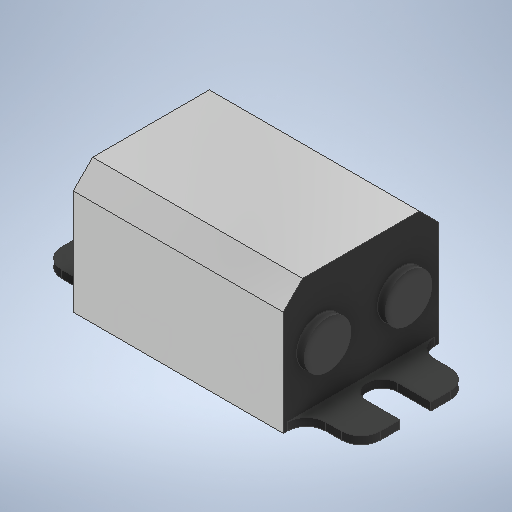
# Autodesk Inventor part: 5vconverter
Saved by Autodesk Inventor 2025 (Build 290162000, 162)
## iProperties
Created: 2025-05-12
Part Number: 5vconverter
Material: Generic
Document SubType Name: Modeling
Designer: ethan
Density: 1 g/cm^3
Appearance: Default
Author: ethan
Autodesk Inventor part; units mm, degrees
ref_plane "YZ Plane" through (0, 0, 0) normal (1, 0, 0) x (0, 1, 0)
ref_plane "XZ Plane" through (0, 0, 0) normal (0, 1, 0) x (-1, 0, 0)
sketch "Sketch1" plane through (0, 0, 0) normal (0, 1, 0) x (-1, 0, 0)
  line L0 (-17.145, 12.7) -> (17.145, 12.7)
  line L1 (17.145, 12.7) -> (17.145, -12.7)
  line L2 (17.145, -12.7) -> (-17.145, -12.7)
  line L3 (-17.145, -12.7) -> (-17.145, 12.7)
  line L4 (-17.145, 12.7) -> (17.145, -12.7) construction
  line L5 (17.145, 12.7) -> (-17.145, -12.7) construction
  point P0 (0, 0)
  dimension "d0" = 34.29
  dimension "d1" = 25.4
  constraints: 12 end point, 2 midpoint, 2 parallel, 1 horizontal, 1 perpendicular
  measures "d0" distance of L1.end L2.end
  measures "d1" distance of L0.end L1.end
extrude "Extrusion1" add sketch "Sketch1" along normal blind 20.32
sketch "Sketch2" plane through (17.145, 0, 12.7) normal (1, 0, 0) x (0, 0, -1)
  line L0 (0, 0) -> (25.4, 0) projected
  line L1 (25.4, 0) -> (25.4, 20.32) projected
  line L2 (0, 20.32) -> (25.4, 20.32) projected
  line L3 (0, 0) -> (0, 20.32) projected
  circle A0 centre (19.2135, 10.16) radius 3.81
  circle A1 centre (5.9899, 10.16) radius 3.81
  point P0 (12.7, 0)
  dimension "d4" = 7.62
  dimension "d5" = 7.62
  constraints: 2 centre point
  measures "d4" diameter of A0
  measures "d5" diameter of A1
ref_plane "Work Plane1" through (0, 0, 12.7) normal (1, 0, 0) x (0, 0, -1)
extrude "Extrusion2" add sketch "Sketch2" along normal blind 1.27 separate body contours A0 | A1
mirror "Mirror1" about plane through (0, 0, 12.7) normal (1, 0, 0) of "Extrusion2" bodies 2
sketch "Sketch3" plane through (0, 0, 0) normal (0, -1, 0) x (1, 0, 0)
  line L0 (17.145, -12.7) -> (-17.145, -12.7) projected
  line L1 (17.145, 12.7) -> (17.145, -12.7) projected
  line L2 (-17.145, 12.7) -> (17.145, 12.7) projected
  line L3 (-17.145, -12.7) -> (-17.145, 12.7) projected
  line L4 (16.1925, 2.54) -> (18.0975, 2.54)
  line L5 (18.0975, 2.54) -> (18.0975, 0)
  line L6 (18.0975, -2.54) -> (16.1925, -2.54)
  line L7 (16.1925, -2.54) -> (16.1925, 2.54)
  line L8 (16.1925, 2.54) -> (18.0975, -2.54) construction
  line L9 (18.0975, 2.54) -> (16.1925, -2.54) construction
  line L10 (20.6375, -2.54) -> (26.035, -2.54)
  line L11 (26.035, -2.54) -> (26.035, -5.715)
  line L12 (22.86, -8.89) -> (20.32, -8.89)
  arc A0 (22.86, -8.89) -> (26.035, -5.715) centre (22.86, -5.715) ccw
  arc A1 (18.0975, 0) -> (20.6375, -2.54) centre (20.6375, 0) ccw
  line L13 (22.86, 0) -> (28.1937, 0)
  line L14 (17.145, 12.7) -> (-17.145, 12.7)
  line L15 (17.145, -12.7) -> (17.145, -12.065)
  line L16 (18.0975, 2.54) -> (16.1925, 2.54)
  line L17 (16.1925, 2.54) -> (16.1925, -2.54)
  line L18 (16.1925, -2.54) -> (18.0975, 2.54) construction
  line L19 (18.0975, -2.54) -> (16.1925, 2.54) construction
  line L20 (20.6375, 2.54) -> (26.035, 2.54)
  line L21 (26.035, 2.54) -> (26.035, 5.715)
  line L22 (22.86, 8.89) -> (20.32, 8.89)
  arc A2 (26.035, 5.715) -> (22.86, 8.89) centre (22.86, 5.715) ccw
  arc A3 (20.6375, 2.54) -> (18.0975, 0) centre (20.6375, 0) ccw
  arc A4 (20.32, -8.89) -> (17.145, -12.065) centre (20.32, -12.065) ccw
  line L23 (17.145, 12.7) -> (17.145, 12.065)
  arc A5 (17.145, 12.065) -> (20.32, 8.89) centre (20.32, 12.065) ccw
  point P0 (0, 0)
  point P1 (17.145, 0)
  point P2 (17.145, -2.54)
  point P3 (26.035, -8.89)
  point P4 (17.145, -8.89)
  point P5 (17.145, 2.54)
  point P6 (26.035, 8.89)
  point P7 (17.145, 8.89)
  dimension "d8" = 1.905
  dimension "d9" = 5.08
  dimension "d10" = 8.89
  dimension "d11" = 6.35
  dimension "d12" = 3.175
  dimension "d13" = 2.54
  dimension "d14" = 3.175
  dimension "d15" = 3.175
  constraints: 40 end point, 15 point on line, 14 symmetric about line, 12 point on circle, 8 tangent, 6 centre point, 4 midpoint, 2 horizontal, 2 parallel, 2 perpendicular, 1 collinear, 1 vertical, 2 other
  measures "d8" distance of L6.start L6.end
  measures "d9" distance of L4.end L6.start
  measures "d10" distance of point (17.145, -2.54) L10.end
  measures "d11" distance of L10.end point (26.035, -8.89)
  measures "d12" radius of A0
  measures "d13" radius of A1
  measures "d14" radius of A4
  measures "d15" radius of A5
extrude "Extrusion3" add sketch "Sketch3" against normal blind 1.27 separate body contours L1 L4 L5 A1 L10 L11 A0 L12 A4 | L1 A5 L22 A2 L21 L20 A3 L5 L4
mirror "Mirror2" about plane through (0, 0, 12.7) normal (1, 0, 0) of "Extrusion3" bodies 3
chamfer "Chamfer1" distance 3.175 angle 45 2 edges at (0, 20.32, 12.7) (0, 20.32, -12.7)
body "Solid1"
body "Solid2"
body "Solid3"
